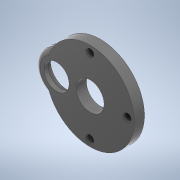
# Autodesk Inventor part: MotorBracket
Saved by Autodesk Inventor 2020 (Build 240168000, 168)
## iProperties
Created: 2019-05-31
Part Number: MotorBracket
Material: ABS Plastic
Document SubType Name: Modeling
Designer: Connor
Density: 1.06 g/cm^3
Appearance: Smooth - Black
Author: Connor
Autodesk Inventor part; units mm, degrees
ref_plane "YZ Plane" through (0, 0, 0) normal (1, 0, 0) x (0, 1, 0)
ref_plane "XZ Plane" through (0, 0, 0) normal (0, 1, 0) x (-1, 0, 0)
ref_plane "XY Plane" through (0, 0, 0) normal (0, 0, 1) x (1, 0, 0)
sketch "Sketch1" plane through (0, 0, 0) normal (0, 0, 1) x (1, 0, 0)
  circle A0 centre (0, 0) radius 11.1125
  circle A1 centre (22.86, 0) radius 9.525
  arc A2 (-3.7868, 13.7765) -> (-3.7868, -13.7765) centre (0, 0) ccw
  circle A3 centre (22.86, -25.4) radius 2.5797
  circle A4 centre (22.86, 0) radius 25.4 construction
  circle A5 centre (48.26, 0) radius 2.5797
  circle A6 centre (22.86, 25.4) radius 2.5797
  circle A7 centre (22.86, 0) radius 29.9974
  dimension "d0" = 22.225
  dimension "d1" = 19.05
  dimension "d2" = 22.86
  dimension "d3" = 3.175
  dimension "d8" = 50.8
  dimension "d11" = 5.1594
  dimension "d17" = 59.9948
  constraints: 8 centre point, 7 point on circle, 3 coincident, 2 equal radius, 2 horizontal alignment, 2 vertical alignment
  measures "d0" diameter of A0
  measures "d1" diameter of A1
  measures "d2" distance of A1.centre point (0, 0)
  measures "d3" radial gap between concentric circles of A0 A2
  measures "d8" diameter of A4
  measures "d11" diameter of A6
  measures "d17" diameter of A7
extrude "Extrusion1" add sketch "Sketch1" along normal blind 6.985 contours A0 A7 | A0 A7 A2 picked at (30.9689, 18.7513)
sketch "Sketch2" plane through (0, 0, 6.985) normal (0, 0, 1) x (1, 0, 0)
  circle A0 centre (0, 0) radius 11.1125 projected
  circle A1 centre (0, 0) radius 8.5725
  dimension "d14" = 2.54
  constraints: 1 centre point
  measures "d14" radial gap between concentric circles of A0 A1
extrude "Extrusion2" add sketch "Sketch2" against normal blind 3.0226
fillet "Fillet1" radius 3.175 1 edges at (-14.2875, 0, 6.985)
body "Solid1"
